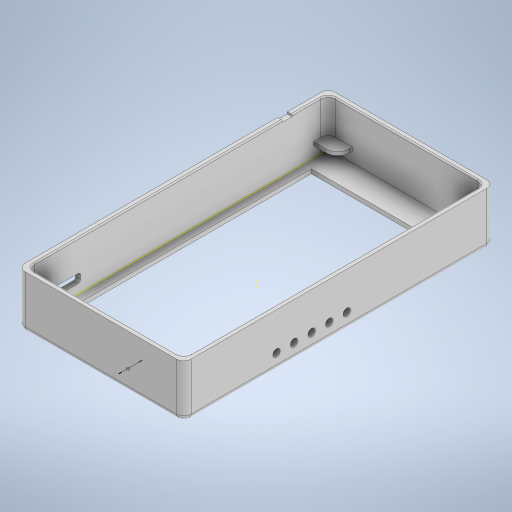
# Autodesk Inventor part: Part3
Saved by Autodesk Inventor 2023 (Build 270158000, 158)
## iProperties
Created: 2022-05-07
Part Number: Part3
Material: Generic
Document SubType Name: Modeling
Designer: filip
Density: 1 g/cm^3
Appearance: Default
Author: filip
Autodesk Inventor part; units mm, degrees
ref_plane "YZ Plane" through (0, 0, 0) normal (1, 0, 0) x (0, 1, 0)
ref_plane "XZ Plane" through (0, 0, 0) normal (0, 1, 0) x (-1, 0, 0)
ref_plane "XY Plane" through (0, 0, 0) normal (0, 0, 1) x (1, 0, 0)
sketch "Sketch1" plane through (0, 0, 0) normal (0, 1, 0) x (-1, 0, 0)
  line L0 (34.5, 64.5) -> (-34.5, 64.5)
  line L1 (-34.5, 64.5) -> (-34.5, -64.5)
  line L2 (-34.5, -64.5) -> (34.5, -64.5)
  line L3 (34.5, -64.5) -> (34.5, 64.5)
  line L4 (34.5, 64.5) -> (-34.5, -64.5) construction
  line L5 (-34.5, 64.5) -> (34.5, -64.5) construction
  point P0 (0, 0)
  dimension "d0" = 69
  dimension "d1" = 129
  constraints: 12 end point, 2 midpoint, 2 parallel, 1 horizontal, 1 perpendicular
  measures "d0" distance of L2.end L1.end
  measures "d1" distance of L0.end L1.end
extrude "Extrusion1" add sketch "Sketch1" along normal blind 1.8
sketch "Sketch2" plane through (0, 1.8, 0) normal (0, 1, 0) x (1, 0, 0)
  line L0 (-29, -52) -> (29, -52)
  line L1 (29, -52) -> (29, 52)
  line L2 (29, 52) -> (-29, 52)
  line L3 (-29, 52) -> (-29, -52)
  line L4 (-29, -52) -> (29, 52) construction
  line L5 (29, -52) -> (-29, 52) construction
  point P0 (0, 0)
  dimension "d4" = 104
  dimension "d5" = 58
  constraints: 12 end point, 2 midpoint, 2 parallel, 1 horizontal, 1 perpendicular
  measures "d4" distance of L0.end L1.end
  measures "d5" distance of L1.end L2.end
extrude "Extrusion2" cut sketch "Sketch2" against normal up to next
sketch "Sketch3" plane through (0, 1.8, 0) normal (0, 1, 0) x (1, 0, 0)
  line L0 (34.5, 64.5) -> (-34.5, 64.5) projected
  line L1 (-34.5, 64.5) -> (34.5, 64.5)
  line L2 (34.5, 64.5) -> (34.5, -64.5)
  line L3 (34.5, -64.5) -> (-34.5, -64.5)
  line L4 (-34.5, -64.5) -> (-34.5, 64.5)
  line L5 (-32.5, 62.5) -> (32.5, 62.5)
  line L6 (32.5, 62.5) -> (32.5, -62.5)
  line L7 (32.5, -62.5) -> (-32.5, -62.5)
  line L8 (-32.5, -62.5) -> (-32.5, 62.5)
  point P0 (0, 0)
  dimension "d8" = 2
  dimension "d9" = 2
  dimension "d10" = 2
  dimension "d11" = 2
  constraints: 16 end point, 4 parallel, 2 horizontal, 2 perpendicular
  measures "d8" distance between parallel lines of L4 L8
  measures "d9" distance between parallel lines of L0 L5
  measures "d10" distance between parallel lines of L6 L2
  measures "d11" distance between parallel lines of L3 L7
extrude "Extrusion3" add sketch "Sketch3" along normal blind 20
sketch "Sketch4" plane through (0, 1.8, 0) normal (0, 1, 0) x (1, 0, 0)
  line L0 (32.5, -62.5) -> (-32.5, -62.5) projected
  line L1 (-32.5, 62.5) -> (-32.5, -62.5) projected
  line L2 (32.5, -62.5) -> (-32.5, -62.5)
  line L3 (-32.5, -62.5) -> (-32.5, -55)
  line L4 (-32.5, -55) -> (32.5, -55)
  line L5 (32.5, -55) -> (32.5, -62.5)
  line L6 (32.5, 62.5) -> (-32.5, 62.5) projected
  dimension "d36" = 117.5
  constraints: 8 end point, 2 parallel, 1 horizontal, 1 perpendicular, 1 point on line
  measures "d36" distance between parallel lines of L4 L6
extrude "Extrusion4" add sketch "Sketch4" along normal blind 3
sketch "Sketch5" plane through (0, 1.8, 0) normal (0, 1, 0) x (1, 0, 0)
  line L0 (-32.5, -62.5) -> (-32.5, 62.5) projected
  line L1 (-32.5, -62) -> (32.5, -62)
  line L2 (32.5, 62.5) -> (32.5, -62.5) projected
  line L3 (29, -52) -> (-29, -52) projected
  point P0 (0, 0)
  dimension "d17" = 10
  constraints: 2 end point, 2 point on line, 1 horizontal
  measures "d17" distance between parallel lines of L3 L1
fillet "Fillet1" radius 3 8 edges at (-32.5, 13.3, 62.5) (-34.5, 10.9, 64.5) (34.5, 10.9, 64.5) (32.5, 13.3, 62.5) (-32.5, 11.8, -62.5) (32.5, 11.8, -62.5) (34.5, 10.9, -64.5) (-34.5, 10.9, -64.5)
fillet "Fillet2" radius 2 8 edges at (33.6213, 0, -63.6213) (0, 0, -64.5) (-33.6213, 0, -63.6213) (-34.5, 0, 0) (-33.6213, 0, 63.6213) (0, 0, 64.5) (33.6213, 0, 63.6213) (34.5, 0, 0)
sketch "Sketch6" plane through (-34.5, 21.8, -61.5) normal (-1, 0, 0) x (0, 0, 1)
  line L0 (6.5, -12) -> (6.5, -15) projected
  line L1 (6.5, -15) -> (6.5, -12) projected
  line L2 (103, -12.7) -> (111, -12.7)
  line L3 (112, -13.7) -> (112, -15.3)
  line L4 (111, -16.3) -> (103, -16.3)
  line L5 (102, -15.3) -> (102, -13.7)
  line L6 (9.5, -20) -> (113.5, -20) projected
  line L7 (113.5, -20) -> (9.5, -20) projected
  line L8 (116.5, -20) -> (2, -20) projected
  line L9 (2, -20) -> (116.5, -20) projected
  arc A0 (103, -12.7) -> (102, -13.7) centre (103, -13.7) ccw
  arc A1 (102, -15.3) -> (103, -16.3) centre (103, -15.3) ccw
  arc A2 (112, -13.7) -> (111, -12.7) centre (111, -13.7) ccw
  arc A3 (111, -16.3) -> (112, -15.3) centre (111, -15.3) ccw
  line L10 (2, -20) -> (-1, -20) projected
  line L11 (-1, -20) -> (2, -20) projected
  line L12 (116.5, -20) -> (116.5, -17)
  point P0 (61.5, -21.8)
  point P1 (102, -12.7)
  point P2 (112, -16.3)
  point P3 (112, -12.7)
  point P4 (121, -15)
  point P5 (112, -14.5)
  point P6 (107, -16.3)
  dimension "d20" = 10
  dimension "d21" = 3.6
  dimension "d25" = 1
  dimension "d38" = 4.5
  dimension "d39" = 3.7
  constraints: 10 end point, 8 point on circle, 8 tangent, 6 point on line, 4 centre point, 3 equal radius, 2 midpoint, 2 parallel, 1 horizontal, 1 perpendicular
  measures "d20" distance of point (102, -12.7) point (112, -12.7)
  measures "d21" distance of point (112, -12.7) point (112, -16.3)
  measures "d25" radius of A0
  measures "d38" horizontal distance of L12.end point (112, -14.5)
  measures "d39" distance from line of point (107, -16.3) L6
extrude "Extrusion5" cut sketch "Sketch6" against normal up to next
sketch "Sketch7" plane through (34.5, 21.8, 61.5) normal (1, 0, 0) x (0, 0, -1)
  line L0 (116.5, -12) -> (116.5, -15) projected
  line L1 (6.5, -20) -> (121, -20) projected
  circle A0 centre (35.5, -15.5) radius 1.5
  line L2 (6.5, -20) -> (6.5, -17) projected
  point P0 (61.5, -21.8)
  point P1 (2, -15)
  point P2 (6.5, -18.5)
  dimension "d29" = 4.5
  dimension "d30" = 3
  dimension "d37" = 29
  constraints: 1 centre point, 1 midpoint, 1 other
  measures "d30" diameter of A0
  measures "d37" horizontal distance of point (6.5, -18.5) A0.centre
extrude "Extrusion6" cut sketch "Sketch7" against normal up to next
pattern_linear "Rectangular Pattern1" count 5 spacing 7.3 along (0, 0, -1) of "Extrusion6"
sketch "Sketch8" plane through (0, 0, 0) normal (0, -1, 0) x (1, 0, 0)
  point P0 (0, 0)
sketch "Sketch9" plane through (-34.5, 21.8, -61.5) normal (-1, 0, 0) x (0, 0, 1)
  line L0 (123, 0) -> (0, 0) projected
  line L1 (14, 0) -> (18, 0)
  line L2 (18, 0) -> (18, -0.75)
  line L3 (18, -0.75) -> (14, -0.75)
  line L4 (14, -0.75) -> (14, 0)
  point P0 (61.5, -21.8)
  point P1 (-1, 0)
  point P2 (14, -0.375)
  point P3 (18, 0)
  dimension "d40" = 0.75
  dimension "d41" = 4
  dimension "d42" = 15
  constraints: 8 end point, 2 parallel, 1 horizontal, 1 midpoint, 1 perpendicular, 1 point on line
  measures "d40" distance between parallel lines of L3 L0
  measures "d41" distance of L2.end L3.end
  measures "d42" horizontal distance of point (14, -0.375) point (-1, 0)
extrude "Extrusion7" cut sketch "Sketch9" against normal up to surface (2 mm away)
fillet "Fillet3" radius 0.5 5 edges at (0, 21.8, 62.5) (-32.5, 21.8, 8) (0, 21.8, -62.5) (-32.5, 21.8, -53.5) (32.5, 21.8, 0)
sketch "Sketch10" plane through (-29.5, 1.8, -62.5) normal (0, 0, 1) x (1, 0, 0)
  line L0 (-3.2949, 5.75) -> (63.1479, 5.75)
  line L1 (63.1479, 5.75) -> (63.1479, 4.25)
  line L2 (63.1479, 4.25) -> (-3.2949, 4.25)
  line L3 (-3.2949, 4.25) -> (-3.2949, 5.75)
  line L4 (59, 0) -> (0, 0) projected
  line L5 (7, 5.75) -> (7, 4.25)
  line L6 (52, 5.75) -> (52, 4.25)
  line L7 (-3, 19.5) -> (-3, 0) projected
  line L8 (62, 0) -> (62, 19.5) projected
  point P0 (29.5, -1.8)
  point P1 (52, 5)
  point P2 (62, 4.25)
  point P3 (62, 5.75)
  point P4 (-3, 5.75)
  point P5 (-3, 4.25)
  dimension "d46" = 4.25
  dimension "d47" = 1.5
  dimension "d48" = 10
  dimension "d49" = 10
  constraints: 12 end point, 4 point on line, 3 perpendicular, 2 parallel, 1 horizontal, 1 midpoint
  measures "d46" distance between parallel lines of L4 L2
  measures "d47" distance between parallel lines of L2 L0
  measures "d48" distance between parallel lines of L7 L5
  measures "d49" distance from line of L8 point (52, 5)
extrude "Extrusion8" add sketch "Sketch10" along normal blind 6 contours L5 L2 L7 L0 | L0 L8 L2 L6
fillet "Fillet4" radius 5 2 edges at (-22.5, 6.8, -56.5) (22.5, 6.8, -56.5)
body "Solid1"
